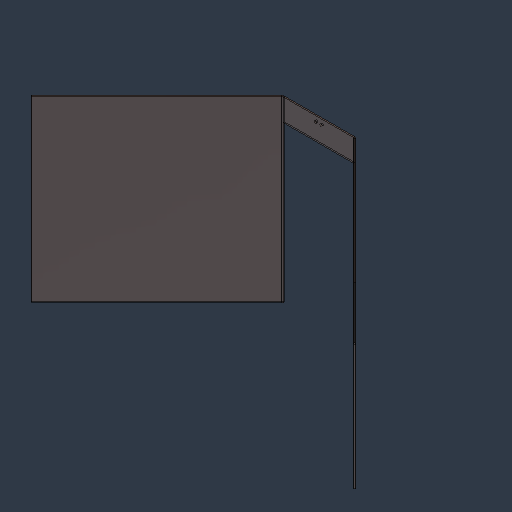
# Autodesk Inventor part: hopper
Saved by Autodesk Inventor 2024.3 (Build 283343000, 343)
## iProperties
Created: 2025-03-05
Part Number: hopper
Material: Polycarbonate, Smoke
Document SubType Name: Sheet Metal
Designer: Marcus Tannini
Density: 1.2 g/cm^3
Sheet Metal Rule: Default
Appearance: Polycarbonate - Smoked
Mass: 1240.94 g
Surface Area: 6892.42 cm^2
Volume: 1034.12 cm^3
Author: Marcus Tannini
Autodesk Inventor part; units mm, degrees
ref_plane "YZ Plane" through (0, 0, 0) normal (1, 0, 0) x (0, 1, 0)
ref_plane "XZ Plane" through (0, 0, 0) normal (0, 1, 0) x (-1, 0, 0)
ref_plane "XY Plane" through (0, 0, 0) normal (0, 0, 1) x (1, 0, 0)
sketch "Sketch1" plane through (0, 0, 0) normal (0, 0, 1) x (1, 0, 0)
  line L0 (-82.55, -203.2) -> (82.55, -203.2)
  line L1 (82.55, -203.2) -> (82.55, 203.2)
  line L2 (82.55, 203.2) -> (-82.55, 203.2)
  line L3 (-82.55, 203.2) -> (-82.55, -203.2)
  line L4 (-82.55, -203.2) -> (82.55, 203.2) construction
  line L5 (82.55, -203.2) -> (-82.55, 203.2) construction
  point P0 (0, 0)
  dimension "d0" = 165.1
  dimension "d1" = 406.4
  measures "d0" distance of L2.end L1.end
  measures "d1" distance of L0.end L1.end
extrude "Plate1" add sketch "Sketch1" along normal blind 3.048
sketch "Sketch2" plane through (80.3947, 203.2, 2.1553) normal (0.7071068, 0, -0.7071068) x (0, 1, 0)
  line L0 (-406.4, 0) -> (0, 0)
  line L1 (0, 0) -> (0, 406.4)
  line L2 (0, 406.4) -> (-406.4, 406.4)
  line L3 (-406.4, 406.4) -> (-406.4, 0)
  constraints: 6 end point, 1 horizontal, 1 perpendicular, 1 vertical
edge flange "Flange1" height 406.4 angle 45 thickness 3.048 bend radius 3.048 thickness toward (0.7071068, 0, -0.7071068) relief straight relief width 3.048 relief depth 1.524 corner gap 3.048 corner form 0 edges at (82.55, 0, 3.048) (-82.55, 0, 3.048) wall of the first edge with corners at (80.3947, -203.2, 2.1553) (80.3947, 203.2, 2.1553) (367.7629, 203.2, 289.5235) (367.7629, -203.2, 289.5235)
bend "Bend1"
corner "Corner1"
sketch "Sketch3" plane through (0, 0, 3.048) normal (0, 0, 1) x (1, 0, 0)
  line L0 (-80.025, 203.2) -> (-80.025, -203.2) construction
  line L1 (80.025, -203.2) -> (-80.025, -203.2) construction
  line L2 (80.025, -203.2) -> (80.025, 203.2) construction
  line L3 (-80.025, 203.2) -> (80.025, 203.2) construction
  line L4 (80.025, -203.2) -> (-80.025, -203.2)
  line L5 (-80.025, -203.2) -> (-80.025, 152.4)
  line L6 (-80.025, 152.4) -> (80.025, 152.4)
  line L7 (80.025, 152.4) -> (80.025, -203.2)
  point P0 (0, 0)
  dimension "d13" = 355.6
  constraints: 8 end point, 2 parallel, 1 horizontal, 1 perpendicular, 1 point on line
  measures "d13" distance of L4.end L5.end
extrude "Cut1" cut sketch "Sketch3" against normal blind 3.048
sketch "Sketch4" plane through (0, 0, 3.048) normal (0, 0, 1) x (1, 0, 0)
  line L0 (-80.025, 152.4) -> (80.025, 152.4) construction
  line L1 (80.025, 152.4) -> (80.025, 203.2) construction
  line L2 (-80.025, 203.2) -> (80.025, 203.2) construction
  line L3 (-80.025, 203.2) -> (-80.025, 152.4) construction
  line L4 (0, 203.2) -> (0, 152.4) construction
  line L5 (0, 190.5) -> (6.35, 190.5)
  point P0 (0, 0)
  point P1 (-6.35, 190.5)
  dimension "d16" = 6.35
  dimension "d17" = 12.7
  constraints: 4 end point, 2 midpoint, 1 coincident, 1 horizontal, 1 point on line, 1 symmetric about line
  measures "d16" distance of L5.start L5.end
  measures "d17" distance between parallel lines of L2 L5
hole "Hole1" at (6.35, 190.5, 3.048) at (-6.35, 190.5, 3.048) direction (0, 0, -1) diameter 5.1054 end through all clearance for "Flat Head Machine Screw (82)" size "#10" standard "Ansi Unified Screw Threads"
equation "\"d14\" = Thickness"
equation "\"d23\" = Thickness"
equation "\"d2\" = Thickness"
equation "\"d3\" = BendReliefWidth"
equation "\"d4\" = BendReliefDepth"
equation "\"d5\" = MinimumRemnant"
equation "\"d6\" = TransitionRadius"
equation "\"d9\" = BendRadius"
equation "\"d10\" = CornerReliefSize"
equation "\"d11\" = GapSize"
equation "\"d12\" = JacobiRadiusSize"
equation "\"BendRadius\" = Thickness"
equation "\"BendReliefWidth\" = Thickness"
equation "\"BendReliefDepth\" = 0.5 * Thickness"
equation "\"CornerReliefSize\" = 4 * Thickness"
equation "\"MinimumRemnant\" = 2 * Thickness"
equation "\"TransitionRadius\" = BendRadius"
equation "\"JacobiRadiusSize\" = BendRadius"
equation "\"GapSize\" = Thickness"
equation "\"Thickness\" = 3.048"
body "Solid1"
